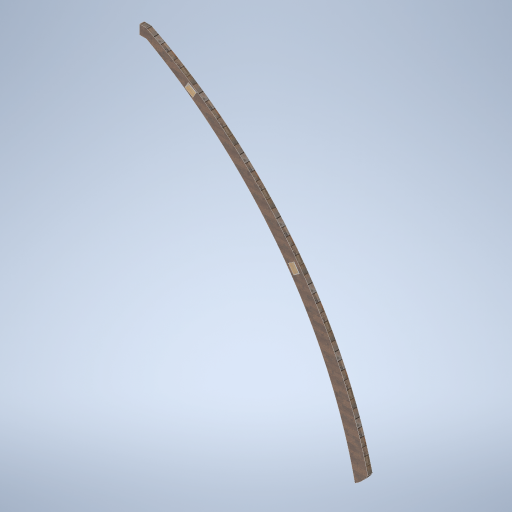
# Autodesk Inventor part: curve_beam_02
Saved by Autodesk Inventor 2024.2 (Build 282272000, 272)
## iProperties
Created: 2024-05-19
Part Number: curve_beam_02
Material: Wood (Maple)
Document SubType Name: Modeling
Designer: LOSTER_1
Density: 0.67 g/cm^3
Appearance: Natural Maple - Glossy Dark Tint
Author: LOSTER_1
Autodesk Inventor part; units mm, degrees
ref_plane "YZ Plane" through (0, 0, 0) normal (1, 0, 0) x (0, 1, 0)
ref_plane "XZ Plane" through (0, 0, 0) normal (0, 1, 0) x (-1, 0, 0)
ref_plane "XY Plane" through (0, 0, 0) normal (0, 0, 1) x (1, 0, 0)
sketch "Sketch1" plane through (0, 0, 0) normal (0, 0, 1) x (1, 0, 0)
  ellipse E0 centre (3487.9501, -1710.9027) end of major axis (3487.9501, -2510.9027) minor radius 800 (3896.5911, -2398.6618) -> (4173.8323, -2122.6862) ccw
  arc A0 (4173.8323, -2122.6862) -> (-553.1987, 3792.9367) centre (-4568.2524, -4261.8348) ccw
  arc A1 (3896.5911, -2398.6618) -> (-553.1987, 3592.9367) centre (-4903.3075, -4285.9308) ccw
  line L0 (-553.1987, 3792.9367) -> (-703.1987, 3792.9367)
  line L1 (-703.1987, 3792.9367) -> (-703.1987, 3592.9367)
  line L2 (-703.1987, 3592.9367) -> (-553.1987, 3592.9367)
  point P0 (0, 0)
  point P1 (3896.5911, -2398.6618)
  point P2 (4173.8323, -2122.6862)
  dimension "d0" = 9000
  dimension "d1" = 9000
  dimension "d2" = 150
  constraints: 6 end point, 4 point on circle, 2 centre point, 2 coincident, 2 perpendicular, 1 horizontal, 4 other
  measures "d0" radius of A0
  measures "d1" radius of A1
  measures "d2" distance of L0.start L0.end
extrude "Extrusion1" add sketch "Sketch1" along normal blind 100
sketch "Sketch2" plane through (0, 0, 100) normal (0, 0, 1) x (1, 0, 0)
  line L0 (264.2908, 3104.5059) -> (437.4958, 3004.5059)
  line L1 (437.4958, 3004.5059) -> (512.4958, 3134.4097)
  line L2 (512.4958, 3134.4097) -> (339.2908, 3234.4097)
  line L3 (339.2908, 3234.4097) -> (264.2908, 3104.5059)
  line L4 (264.2908, 3104.5059) -> (512.4958, 3134.4097) construction
  line L5 (437.4958, 3004.5059) -> (339.2908, 3234.4097) construction
  line L6 (264.2908, 3104.5059) -> (464.2908, 3104.5059) construction
  line L7 (2475.0978, 959.4308) -> (2589.8131, 795.6004)
  line L8 (2589.8131, 795.6004) -> (2712.6859, 881.6369)
  line L9 (2712.6859, 881.6369) -> (2597.9706, 1045.4673)
  line L10 (2597.9706, 1045.4673) -> (2475.0978, 959.4308)
  line L11 (2475.0978, 959.4308) -> (2712.6859, 881.6369) construction
  line L12 (2589.8131, 795.6004) -> (2597.9706, 1045.4673) construction
  line L13 (2475.0978, 959.4308) -> (2675.0978, 959.4308) construction
  point P0 (0, 0)
  point P1 (388.3933, 3119.4578)
  point P2 (2593.8918, 920.5338)
  dimension "d5" = 200
  dimension "d6" = 30
  dimension "d7" = 150
  dimension "d8" = 200
  dimension "d9" = 55
  dimension "d10" = 150
  constraints: 28 end point, 4 midpoint, 4 parallel, 2 equal length, 2 horizontal, 2 perpendicular
  measures "d5" distance of L0.start L0.end
  measures "d6" angle of L0 L6
  measures "d7" distance of L1.end L0.end
  measures "d8" distance of L7.start L7.end
  measures "d9" angle of L7 L13
  measures "d10" distance of L8.end L7.end
extrude "Extrusion2" cut sketch "Sketch2" against normal through all
body "Solid1"
